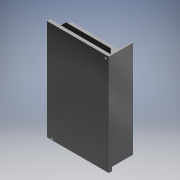
# Autodesk Inventor part: source
Saved by Autodesk Inventor 2018 (Build 220112000, 112)
## iProperties
Created: 2018-05-21
Part Number: source
Material: Generic
Document SubType Name: Modeling
Designer: David
Density: 1 g/cm^3
Appearance: Default
Author: David
Autodesk Inventor part; units mm, degrees
ref_plane "YZ Plane" through (0, 0, 0) normal (1, 0, 0) x (0, 1, 0)
ref_plane "XZ Plane" through (0, 0, 0) normal (0, 1, 0) x (-1, 0, 0)
ref_plane "XY Plane" through (0, 0, 0) normal (0, 0, 1) x (1, 0, 0)
sketch "Sketch1" plane through (0, 0, 0) normal (0, 1, 0) x (-1, 0, 0)
  line L0 (-48.5, -79) -> (48.5, -79)
  line L1 (48.5, -79) -> (48.5, 79)
  line L2 (48.5, 79) -> (-48.5, 79)
  line L3 (-48.5, 79) -> (-48.5, -79)
  line L4 (-48.5, -79) -> (48.5, 79) construction
  line L5 (48.5, -79) -> (-48.5, 79) construction
  point P0 (0, 0)
  dimension "d0" = 97
  dimension "d1" = 158
  constraints: 12 end point, 2 midpoint, 2 parallel, 1 horizontal, 1 perpendicular
  measures "d0" distance of L2.end L1.end
  measures "d1" distance of L1.end L0.end
extrude "Extrusion1" add sketch "Sketch1" along normal blind 5
sketch "Sketch2" plane through (0, 5, 0) normal (0, 1, 0) x (1, 0, 0)
  circle A0 centre (-41, 76.75) radius 1.75
  line L0 (-48.5, -79) -> (48.5, -79) projected
  line L1 (48.5, -79) -> (48.5, 79) projected
  circle A1 centre (43.5, -74.5) radius 1.75
  point P0 (0, 0)
  dimension "d4" = 3.5
  dimension "d5" = 155.75
  dimension "d6" = 89.5
  dimension "d7" = 3.5
  dimension "d8" = 4.5
  dimension "d9" = 5
  constraints: 2 centre point
  measures "d4" diameter of A0
  measures "d5" distance from line of L0 A0.centre
  measures "d6" distance from line of L1 A0.centre
  measures "d7" diameter of A1
  measures "d8" distance from line of L0 A1.centre
  measures "d9" distance from line of L1 A1.centre
extrude "Extrusion2" cut sketch "Sketch2" against normal blind 5
sketch "Sketch3" plane through (0, 5, 0) normal (0, 1, 0) x (1, 0, 0)
  line L0 (48.5, -79) -> (48.5, 79) projected
  line L1 (-48.5, 79) -> (-48.5, -79) projected
  line L2 (48.5, 73) -> (-48.5, 73)
  line L3 (-48.5, 73) -> (-48.5, -59)
  line L4 (-48.5, -59) -> (48.5, -59)
  line L5 (48.5, -59) -> (48.5, 73)
  line L6 (48.5, 79) -> (-48.5, 79) projected
  line L7 (-48.5, -79) -> (48.5, -79) projected
  point P0 (0, 0)
  dimension "d12" = 6
  dimension "d13" = 20
  constraints: 8 end point, 2 parallel, 2 point on line, 1 horizontal, 1 perpendicular
  measures "d12" distance between parallel lines of L2 L6
  measures "d13" distance between parallel lines of L7 L4
extrude "Extrusion3" add sketch "Sketch3" along normal blind 33 contours L4 L1 L2 L0
sketch "Sketch4" plane through (-48.5, 5, 59) normal (0, 0, 1) x (1, 0, 0)
  line L0 (0, 33) -> (97, 33) projected
  line L1 (97, 0) -> (0, 0) projected
  line L2 (97, 33) -> (95, 33)
  line L3 (95, 33) -> (95, 0)
  line L4 (95, 0) -> (97, 0)
  line L5 (97, 0) -> (97, 33)
  point P0 (48.5, -5)
  dimension "d16" = 2
  constraints: 8 end point, 2 parallel, 1 horizontal, 1 perpendicular, 1 point on line
  measures "d16" distance of L4.end L3.end
extrude "Extrusion4" add sketch "Sketch4" along normal blind 20
sketch "Sketch5" plane through (0, 5, 0) normal (0, 1, 0) x (1, 0, 0)
  line L0 (31.5, -59) -> (-38.5, -59)
  line L1 (-38.5, -59) -> (-38.5, -72)
  line L2 (-38.5, -72) -> (31.5, -72)
  line L3 (31.5, -72) -> (31.5, -59)
  line L4 (-48.5, -59) -> (-48.5, -79) projected
  line L5 (46.5, -59) -> (-48.5, -59) projected
  line L6 (-48.5, -79) -> (46.5, -79) projected
  point P0 (0, 0)
  dimension "d19" = 70
  dimension "d20" = 10
  dimension "d21" = 7
  constraints: 8 end point, 2 parallel, 1 collinear, 1 horizontal, 1 perpendicular
  measures "d19" distance of L2.end L1.end
  measures "d20" distance between parallel lines of L4 L1
  measures "d21" distance between parallel lines of L6 L2
extrude "Extrusion5" add sketch "Sketch5" along normal blind 15
body "Solid1"
